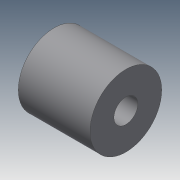
# Autodesk Inventor part: DR-30-6,35x10
Saved by Autodesk Inventor 2016 SP1 (Build 200210100, 210)
## iProperties
Company: Проектная группа
Created: 2017-01-31
Part Number: DR-30-6,35x10
Checked By: Сидоров ИА
Engr Approved By: Баев БГ
Material: Типовые
Document SubType Name: Modeling
Mfg Approved By: Босов АА
Designer: t1
Engineer: Иванов НИ
Authority: Петров ПП
Mass: 19.5526 g
Surface Area: 49.4829 cm^2
Volume: 19.5526 cm^3
Density: 1 g/cm^3
Appearance: По умолчанию
Author: t1
Autodesk Inventor part; units mm, degrees
ref_plane "YZ Plane" through (0, 0, 0) normal (1, 0, 0) x (0, 1, 0)
ref_plane "XZ Plane" through (0, 0, 0) normal (0, 1, 0) x (-1, 0, 0)
ref_plane "XY Plane" through (0, 0, 0) normal (0, 0, 1) x (1, 0, 0)
sketch "Эскиз3" plane through (0, 0, 0) normal (0, 0, 1) x (1, 0, 0)
  line L0 (-20.1552, 0) -> (30.6288, 0)
  line L1 (15, 15) -> (12, 15)
  line L2 (15, 5) -> (15, 15)
  line L3 (-4, 3.175) -> (-15, 3.175)
  line L4 (-15, 3.175) -> (-15, 15)
  line L5 (4, 5) -> (15, 5)
  line L6 (-30.312, 0) -> (40.7856, 0) projected
  line L7 (4, 5) -> (0, 5)
  line L8 (0, 5) -> (0, 3.175)
  line L9 (0, 3.175) -> (-4, 3.175)
  line L10 (12, 15) -> (-15, 15)
  dimension "d43" = 6.35
  dimension "d50" = 30
  dimension "d51" = 10
  dimension "d61" = 30
  constraints: 20 end point, 6 perpendicular, 3 horizontal, 1 collinear, 1 parallel
  measures "d43" diameter of L3 L0
  measures "d50" distance between parallel lines of L2 L4
  measures "d51" diameter of L5 L0
  measures "d61" diameter of L10 L0
revolve "Вращение5" add sketch "Эскиз3" angle 360 about axis through (-20.1552, 0, 0) along (1, 0, 0)
